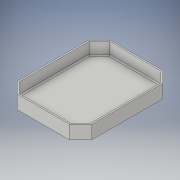
# Autodesk Inventor part: Kozhuh_Lock
Saved by Autodesk Inventor 2017 (Build 210142000, 142)
## iProperties
Part Number: Kozhuh_Lock
Material: Типовые
Document SubType Name: Modeling
Designer: yulia_000
Density: 1 g/cm^3
Appearance: По умолчанию
Author: yulia_000
Autodesk Inventor part; units mm, degrees
ref_plane "YZ Plane" through (0, 0, 0) normal (1, 0, 0) x (0, 1, 0)
ref_plane "XZ Plane" through (0, 0, 0) normal (0, 1, 0) x (-1, 0, 0)
ref_plane "XY Plane" through (0, 0, 0) normal (0, 0, 1) x (1, 0, 0)
sketch "Эскиз1" plane through (0, 0, 0) normal (0, 1, 0) x (-1, 0, 0)
  line L0 (8.5, 0) -> (50.1, 0)
  line L1 (58.6, -8.5) -> (58.6, -65.5)
  line L2 (50.1, -74) -> (8.5, -74)
  line L3 (0, -65.5) -> (0, -8.5)
  line L4 (58.6, -8.5) -> (50.1, 0)
  line L5 (58.6, -65.5) -> (50.1, -74)
  line L6 (8.5, -74) -> (0, -65.5)
  line L7 (0, -8.5) -> (8.5, 0)
  line L8 (59.8, -65.9971) -> (50.5971, -75.2)
  line L9 (50.5971, -75.2) -> (8.0029, -75.2)
  line L10 (8.0029, -75.2) -> (-1.2, -65.9971)
  line L11 (-1.2, -65.9971) -> (-1.2, -8.0029)
  line L12 (-1.2, -8.0029) -> (8.0029, 1.2)
  line L13 (8.0029, 1.2) -> (50.5971, 1.2)
  line L14 (50.5971, 1.2) -> (59.8, -8.0029)
  line L15 (59.8, -8.0029) -> (59.8, -65.9971)
  point P0 (0, 0)
  point P1 (58.6, -74)
  point P2 (58.6, 0)
  point P3 (0, -74)
  dimension "d8" = 58.6
  dimension "d9" = 74
  dimension "d10" = 8.5
  dimension "d11" = 8.5
  dimension "d12" = 8.5
  dimension "d13" = 8.5
  dimension "d14" = 8.5
  dimension "d15" = 8.5
  dimension "d16" = 8.5
  dimension "d17" = 8.5
  dimension "d18" = 1.2
  constraints: 32 end point, 8 point on line, 4 parallel, 2 perpendicular, 1 horizontal, 7 other
  measures "d8" distance of point (58.6, -74) point (0, -74)
  measures "d9" distance of point (58.6, 0) point (58.6, -74)
  measures "d10" distance of L1.start point (58.6, 0)
  measures "d11" distance of L0.end point (58.6, 0)
  measures "d12" distance of L1.end point (58.6, -74)
  measures "d13" distance of L2.start point (58.6, -74)
  measures "d14" distance of L2.end point (0, -74)
  measures "d15" distance of L3.start point (0, -74)
  measures "d16" distance of L3.end point (0, 0)
  measures "d17" distance of L0.start point (0, 0)
  measures "d18" distance between parallel lines of L1 L15
extrude "Выдавливание1" add sketch "Эскиз1" against normal blind 1 contours L0 L4 L1 L5 L2 L6 L3 L7 | L8 L9 L10 L11 L12 L13 L14 L15
extrude "Выдавливание2" add sketch "Эскиз1" along normal blind 10
fillet "Сопряжение1" radius 1 8 edges at (-58.6, 0, -37) (-54.35, 0, -69.75) (-29.3, 0, -74) (-4.25, 0, -69.75) (0, 0, -37) (-4.25, 0, -4.25) (-29.3, 0, 0) (-54.35, 0, -4.25)
equation "\"d11\" = d10"
equation "\"d12\" = d10"
equation "\"d13\" = d12"
equation "\"d14\" = d10"
equation "\"d15\" = d14"
equation "\"d16\" = d10"
equation "\"d17\" = d16"
